Autodesk Inventor part; units mm, degrees
(part 2 of 7)
  line L132 (47.0881, -59.4916) -> (33.6537, -59.4916)
  arc A151 (44.1532, -52.5346) -> (44.1532, -56.5346) centre (44.1532, -54.5346) ccw
  line L133 (57.5876, -52.5346) -> (44.1532, -52.5346)
  arc A152 (57.5876, -56.5346) -> (57.5876, -52.5346) centre (57.5876, -54.5346) ccw
  line L134 (44.1532, -56.5346) -> (57.5876, -56.5346)
  line L135 (13.6537, -63.4916) -> (27.0881, -63.4916)
  line L136 (27.0881, -59.4916) -> (13.6537, -59.4916)
  arc A153 (24.1532, -52.5346) -> (24.1532, -56.5346) centre (24.1532, -54.5346) ccw
  arc A154 (27.0881, -63.4916) -> (27.0881, -59.4916) centre (27.0881, -61.4916) ccw
  arc A155 (33.6537, -59.4916) -> (33.6537, -63.4916) centre (33.6537, -61.4916) ccw
  line L137 (37.5876, -52.5346) -> (24.1532, -52.5346)
  line L138 (24.1532, -56.5346) -> (37.5876, -56.5346)
  arc A156 (37.5876, -56.5346) -> (37.5876, -52.5346) centre (37.5876, -54.5346) ccw
  line L139 (33.6537, -63.4916) -> (47.0881, -63.4916)
  arc A157 (-6.3463, -59.4916) -> (-6.3463, -63.4916) centre (-6.3463, -61.4916) ccw
  arc A158 (27.0881, -63.4916) -> (27.0881, -59.4916) centre (27.0881, -61.4916) ccw
  arc A159 (24.1532, -52.5346) -> (24.1532, -56.5346) centre (24.1532, -54.5346) ccw
  line L140 (27.0881, -59.4916) -> (13.6537, -59.4916)
  arc A160 (24.1532, -52.5346) -> (24.1532, -56.5346) centre (24.1532, -54.5346) ccw
  line L141 (37.5876, -52.5346) -> (24.1532, -52.5346)
  arc A161 (37.5876, -56.5346) -> (37.5876, -52.5346) centre (37.5876, -54.5346) ccw
  line L142 (24.1532, -56.5346) -> (37.5876, -56.5346)
  line L143 (-6.3463, -63.4916) -> (7.0881, -63.4916)
  line L144 (7.0881, -59.4916) -> (-6.3463, -59.4916)
  arc A162 (4.1532, -52.5346) -> (4.1532, -56.5346) centre (4.1532, -54.5346) ccw
  arc A163 (7.0881, -63.4916) -> (7.0881, -59.4916) centre (7.0881, -61.4916) ccw
  arc A164 (13.6537, -59.4916) -> (13.6537, -63.4916) centre (13.6537, -61.4916) ccw
  line L145 (17.5876, -52.5346) -> (4.1532, -52.5346)
  line L146 (4.1532, -56.5346) -> (17.5876, -56.5346)
  arc A165 (17.5876, -56.5346) -> (17.5876, -52.5346) centre (17.5876, -54.5346) ccw
  line L147 (13.6537, -63.4916) -> (27.0881, -63.4916)
  arc A166 (-26.3463, -59.4916) -> (-26.3463, -63.4916) centre (-26.3463, -61.4916) ccw
  arc A167 (7.0881, -63.4916) -> (7.0881, -59.4916) centre (7.0881, -61.4916) ccw
  arc A168 (4.1532, -52.5346) -> (4.1532, -56.5346) centre (4.1532, -54.5346) ccw
  line L148 (7.0881, -59.4916) -> (-6.3463, -59.4916)
  arc A169 (4.1532, -52.5346) -> (4.1532, -56.5346) centre (4.1532, -54.5346) ccw
  line L149 (17.5876, -52.5346) -> (4.1532, -52.5346)
  arc A170 (17.5876, -56.5346) -> (17.5876, -52.5346) centre (17.5876, -54.5346) ccw
  line L150 (4.1532, -56.5346) -> (17.5876, -56.5346)
  line L151 (-26.3463, -63.4916) -> (-12.9119, -63.4916)
  line L152 (-12.9119, -59.4916) -> (-26.3463, -59.4916)
  arc A171 (-15.8468, -52.5346) -> (-15.8468, -56.5346) centre (-15.8468, -54.5346) ccw
  arc A172 (-12.9119, -63.4916) -> (-12.9119, -59.4916) centre (-12.9119, -61.4916) ccw
  arc A173 (-6.3463, -59.4916) -> (-6.3463, -63.4916) centre (-6.3463, -61.4916) ccw
  line L153 (-2.4124, -52.5346) -> (-15.8468, -52.5346)
  line L154 (-15.8468, -56.5346) -> (-2.4124, -56.5346)
  arc A174 (-2.4124, -56.5346) -> (-2.4124, -52.5346) centre (-2.4124, -54.5346) ccw
  line L155 (-6.3463, -63.4916) -> (7.0881, -63.4916)
  arc A175 (-46.3463, -59.4916) -> (-46.3463, -63.4916) centre (-46.3463, -61.4916) ccw
  arc A176 (-12.9119, -63.4916) -> (-12.9119, -59.4916) centre (-12.9119, -61.4916) ccw
  arc A177 (-15.8468, -52.5346) -> (-15.8468, -56.5346) centre (-15.8468, -54.5346) ccw
  line L156 (-12.9119, -59.4916) -> (-26.3463, -59.4916)
  arc A178 (-15.8468, -52.5346) -> (-15.8468, -56.5346) centre (-15.8468, -54.5346) ccw
  line L157 (-2.4124, -52.5346) -> (-15.8468, -52.5346)
  arc A179 (-2.4124, -56.5346) -> (-2.4124, -52.5346) centre (-2.4124, -54.5346) ccw
  line L158 (-15.8468, -56.5346) -> (-2.4124, -56.5346)
  line L159 (-46.3463, -63.4916) -> (-32.9119, -63.4916)
  line L160 (-32.9119, -59.4916) -> (-46.3463, -59.4916)
  arc A180 (-35.8468, -52.5346) -> (-35.8468, -56.5346) centre (-35.8468, -54.5346) ccw
  arc A181 (-32.9119, -63.4916) -> (-32.9119, -59.4916) centre (-32.9119, -61.4916) ccw
  arc A182 (-26.3463, -59.4916) -> (-26.3463, -63.4916) centre (-26.3463, -61.4916) ccw
  line L161 (-22.4124, -52.5346) -> (-35.8468, -52.5346)
  line L162 (-35.8468, -56.5346) -> (-22.4124, -56.5346)
  arc A183 (-22.4124, -56.5346) -> (-22.4124, -52.5346) centre (-22.4124, -54.5346) ccw
  line L163 (-26.3463, -63.4916) -> (-12.9119, -63.4916)
  arc A184 (-66.3463, -59.4916) -> (-66.3463, -63.4916) centre (-66.3463, -61.4916) ccw
  arc A185 (-32.9119, -63.4916) -> (-32.9119, -59.4916) centre (-32.9119, -61.4916) ccw
  arc A186 (-35.8468, -52.5346) -> (-35.8468, -56.5346) centre (-35.8468, -54.5346) ccw
  line L164 (-32.9119, -59.4916) -> (-46.3463, -59.4916)
  arc A187 (-35.8468, -52.5346) -> (-35.8468, -56.5346) centre (-35.8468, -54.5346) ccw
  line L165 (-22.4124, -52.5346) -> (-35.8468, -52.5346)
  arc A188 (-22.4124, -56.5346) -> (-22.4124, -52.5346) centre (-22.4124, -54.5346) ccw
  line L166 (-35.8468, -56.5346) -> (-22.4124, -56.5346)
  line L167 (-66.3463, -63.4916) -> (-52.9119, -63.4916)
  line L168 (-52.9119, -59.4916) -> (-66.3463, -59.4916)
  arc A189 (-55.8468, -52.5346) -> (-55.8468, -56.5346) centre (-55.8468, -54.5346) ccw
  arc A190 (-52.9119, -63.4916) -> (-52.9119, -59.4916) centre (-52.9119, -61.4916) ccw
  arc A191 (-46.3463, -59.4916) -> (-46.3463, -63.4916) centre (-46.3463, -61.4916) ccw
  line L169 (-42.4124, -52.5346) -> (-55.8468, -52.5346)
  line L170 (-55.8468, -56.5346) -> (-42.4124, -56.5346)
  arc A192 (-42.4124, -56.5346) -> (-42.4124, -52.5346) centre (-42.4124, -54.5346) ccw
  line L171 (-46.3463, -63.4916) -> (-32.9119, -63.4916)
  arc A193 (44.1532, -38.5346) -> (44.1532, -42.5346) centre (44.1532, -40.5346) ccw
  arc A194 (44.1532, -38.5346) -> (44.1532, -42.5346) centre (44.1532, -40.5346) ccw
  arc A195 (44.1532, -38.5346) -> (44.1532, -42.5346) centre (44.1532, -40.5346) ccw
  arc A196 (44.1532, -38.5346) -> (44.1532, -42.5346) centre (44.1532, -40.5346) ccw
  arc A197 (44.1532, -38.5346) -> (44.1532, -42.5346) centre (44.1532, -40.5346) ccw
  arc A198 (44.1532, -38.5346) -> (44.1532, -42.5346) centre (44.1532, -40.5346) ccw
  arc A199 (44.1532, -38.5346) -> (44.1532, -42.5346) centre (44.1532, -40.5346) ccw
  arc A200 (33.6537, -45.4916) -> (33.6537, -49.4916) centre (33.6537, -47.4916) ccw
  arc A201 (27.0881, -49.4916) -> (27.0881, -45.4916) centre (27.0881, -47.4916) ccw
  arc A202 (27.0881, -49.4916) -> (27.0881, -45.4916) centre (27.0881, -47.4916) ccw
  arc A203 (33.6537, -45.4916) -> (33.6537, -49.4916) centre (33.6537, -47.4916) ccw
  arc A204 (27.0881, -49.4916) -> (27.0881, -45.4916) centre (27.0881, -47.4916) ccw
  arc A205 (27.0881, -49.4916) -> (27.0881, -45.4916) centre (27.0881, -47.4916) ccw
  arc A206 (27.0881, -49.4916) -> (27.0881, -45.4916) centre (27.0881, -47.4916) ccw
  arc A207 (27.0881, -49.4916) -> (27.0881, -45.4916) centre (27.0881, -47.4916) ccw
  arc A208 (33.6537, -45.4916) -> (33.6537, -49.4916) centre (33.6537, -47.4916) ccw
  arc A209 (33.6537, -45.4916) -> (33.6537, -49.4916) centre (33.6537, -47.4916) ccw
  arc A210 (33.6537, -45.4916) -> (33.6537, -49.4916) centre (33.6537, -47.4916) ccw
  line L172 (24.1532, -42.5346) -> (37.5876, -42.5346)
  line L173 (37.5876, -38.5346) -> (24.1532, -38.5346)
  line L174 (24.1532, -42.5346) -> (37.5876, -42.5346)
  line L175 (24.1532, -42.5346) -> (37.5876, -42.5346)
  line L176 (24.1532, -42.5346) -> (37.5876, -42.5346)
  line L177 (24.1532, -42.5346) -> (37.5876, -42.5346)
  line L178 (24.1532, -42.5346) -> (37.5876, -42.5346)
  line L179 (37.5876, -38.5346) -> (24.1532, -38.5346)
  line L180 (37.5876, -38.5346) -> (24.1532, -38.5346)
  line L181 (37.5876, -38.5346) -> (24.1532, -38.5346)
  line L182 (37.5876, -38.5346) -> (24.1532, -38.5346)
  line L183 (37.5876, -38.5346) -> (24.1532, -38.5346)
  arc A211 (37.5876, -42.5346) -> (37.5876, -38.5346) centre (37.5876, -40.5346) ccw
  arc A212 (37.5876, -42.5346) -> (37.5876, -38.5346) centre (37.5876, -40.5346) ccw
  arc A213 (37.5876, -42.5346) -> (37.5876, -38.5346) centre (37.5876, -40.5346) ccw
  arc A214 (37.5876, -42.5346) -> (37.5876, -38.5346) centre (37.5876, -40.5346) ccw
  arc A215 (37.5876, -42.5346) -> (37.5876, -38.5346) centre (37.5876, -40.5346) ccw
  arc A216 (37.5876, -42.5346) -> (37.5876, -38.5346) centre (37.5876, -40.5346) ccw
  arc A217 (44.1532, -38.5346) -> (44.1532, -42.5346) centre (44.1532, -40.5346) ccw
  arc A218 (47.0881, -49.4916) -> (47.0881, -45.4916) centre (47.0881, -47.4916) ccw
  arc A219 (47.0881, -49.4916) -> (47.0881, -45.4916) centre (47.0881, -47.4916) ccw
  arc A220 (53.6537, -45.4916) -> (53.6537, -49.4916) centre (53.6537, -47.4916) ccw
  arc A221 (47.0881, -49.4916) -> (47.0881, -45.4916) centre (47.0881, -47.4916) ccw
  arc A222 (47.0881, -49.4916) -> (47.0881, -45.4916) centre (47.0881, -47.4916) ccw
  arc A223 (47.0881, -49.4916) -> (47.0881, -45.4916) centre (47.0881, -47.4916) ccw
  arc A224 (53.6537, -45.4916) -> (53.6537, -49.4916) centre (53.6537, -47.4916) ccw
  arc A225 (53.6537, -45.4916) -> (53.6537, -49.4916) centre (53.6537, -47.4916) ccw
  line L184 (57.5876, -38.5346) -> (44.1532, -38.5346)
  line L185 (44.1532, -42.5346) -> (57.5876, -42.5346)
  line L186 (57.5876, -38.5346) -> (44.1532, -38.5346)
  line L187 (44.1532, -42.5346) -> (57.5876, -42.5346)
  line L188 (44.1532, -42.5346) -> (57.5876, -42.5346)
  line L189 (44.1532, -42.5346) -> (57.5876, -42.5346)
  line L190 (44.1532, -42.5346) -> (57.5876, -42.5346)
  line L191 (57.5876, -38.5346) -> (44.1532, -38.5346)
  line L192 (57.5876, -38.5346) -> (44.1532, -38.5346)
  line L193 (57.5876, -38.5346) -> (44.1532, -38.5346)
  arc A226 (57.5876, -42.5346) -> (57.5876, -38.5346) centre (57.5876, -40.5346) ccw
  arc A227 (64.1532, -38.5346) -> (64.1532, -42.5346) centre (64.1532, -40.5346) ccw
  line L194 (53.6537, -49.4916) -> (67.0881, -49.4916)
  line L195 (53.6537, -49.4916) -> (67.0881, -49.4916)
  line L196 (53.6537, -49.4916) -> (67.0881, -49.4916)
  line L197 (67.0881, -45.4916) -> (53.6537, -45.4916)
  line L198 (67.0881, -45.4916) -> (53.6537, -45.4916)
  line L199 (67.0881, -45.4916) -> (53.6537, -45.4916)
  arc A228 (64.1532, -38.5346) -> (64.1532, -42.5346) centre (64.1532, -40.5346) ccw
  arc A229 (64.1532, -38.5346) -> (64.1532, -42.5346) centre (64.1532, -40.5346) ccw
  arc A230 (64.1532, -38.5346) -> (64.1532, -42.5346) centre (64.1532, -40.5346) ccw
  arc A231 (64.1532, -38.5346) -> (64.1532, -42.5346) centre (64.1532, -40.5346) ccw
  arc A232 (57.5876, -42.5346) -> (57.5876, -38.5346) centre (57.5876, -40.5346) ccw
  arc A233 (57.5876, -42.5346) -> (57.5876, -38.5346) centre (57.5876, -40.5346) ccw
  arc A234 (57.5876, -42.5346) -> (57.5876, -38.5346) centre (57.5876, -40.5346) ccw
  arc A235 (57.5876, -42.5346) -> (57.5876, -38.5346) centre (57.5876, -40.5346) ccw
  arc A236 (67.0881, -49.4916) -> (67.0881, -45.4916) centre (67.0881, -47.4916) ccw
  arc A237 (67.0881, -49.4916) -> (67.0881, -45.4916) centre (67.0881, -47.4916) ccw
  arc A238 (67.0881, -49.4916) -> (67.0881, -45.4916) centre (67.0881, -47.4916) ccw
  line L200 (77.5876, -38.5346) -> (64.1532, -38.5346)
  line L201 (77.5876, -38.5346) -> (64.1532, -38.5346)
  line L202 (77.5876, -38.5346) -> (64.1532, -38.5346)
  line L203 (64.1532, -42.5346) -> (77.5876, -42.5346)
  line L204 (64.1532, -42.5346) -> (77.5876, -42.5346)
  line L205 (64.1532, -42.5346) -> (77.5876, -42.5346)
  arc A239 (73.6537, -45.4916) -> (73.6537, -49.4916) centre (73.6537, -47.4916) ccw
  arc A240 (77.5876, -42.5346) -> (77.5876, -38.5346) centre (77.5876, -40.5346) ccw
  arc A241 (77.5876, -42.5346) -> (77.5876, -38.5346) centre (77.5876, -40.5346) ccw
  arc A242 (77.5876, -42.5346) -> (77.5876, -38.5346) centre (77.5876, -40.5346) ccw
  arc A243 (84.1532, -38.5346) -> (84.1532, -42.5346) centre (84.1532, -40.5346) ccw
  arc A244 (84.1532, -38.5346) -> (84.1532, -42.5346) centre (84.1532, -40.5346) ccw
  line L206 (87.0881, -45.4916) -> (73.6537, -45.4916)
  arc A245 (87.0881, -49.4916) -> (87.0881, -45.4916) centre (87.0881, -47.4916) ccw
  line L207 (73.6537, -49.4916) -> (87.0881, -49.4916)
  line L208 (84.1532, -42.5346) -> (97.5876, -42.5346)
  line L209 (97.5876, -38.5346) -> (84.1532, -38.5346)
  arc A246 (97.5876, -42.5346) -> (97.5876, -38.5346) centre (97.5876, -40.5346) ccw
  line L210 (33.6537, -49.4916) -> (47.0881, -49.4916)
  line L211 (47.0881, -45.4916) -> (33.6537, -45.4916)
  line L212 (33.6537, -49.4916) -> (47.0881, -49.4916)
  line L213 (47.0881, -45.4916) -> (33.6537, -45.4916)
  line L214 (47.0881, -45.4916) -> (33.6537, -45.4916)
  line L215 (47.0881, -45.4916) -> (33.6537, -45.4916)
  line L216 (47.0881, -45.4916) -> (33.6537, -45.4916)
  line L217 (33.6537, -49.4916) -> (47.0881, -49.4916)
  line L218 (33.6537, -49.4916) -> (47.0881, -49.4916)
  line L219 (33.6537, -49.4916) -> (47.0881, -49.4916)
  arc A247 (13.6537, -45.4916) -> (13.6537, -49.4916) centre (13.6537, -47.4916) ccw
  arc A248 (13.6537, -45.4916) -> (13.6537, -49.4916) centre (13.6537, -47.4916) ccw
  arc A249 (13.6537, -45.4916) -> (13.6537, -49.4916) centre (13.6537, -47.4916) ccw
  arc A250 (13.6537, -45.4916) -> (13.6537, -49.4916) centre (13.6537, -47.4916) ccw
  arc A251 (13.6537, -45.4916) -> (13.6537, -49.4916) centre (13.6537, -47.4916) ccw
  arc A252 (13.6537, -45.4916) -> (13.6537, -49.4916) centre (13.6537, -47.4916) ccw
  arc A253 (7.0881, -49.4916) -> (7.0881, -45.4916) centre (7.0881, -47.4916) ccw
  arc A254 (7.0881, -49.4916) -> (7.0881, -45.4916) centre (7.0881, -47.4916) ccw
  arc A255 (7.0881, -49.4916) -> (7.0881, -45.4916) centre (7.0881, -47.4916) ccw
  arc A256 (7.0881, -49.4916) -> (7.0881, -45.4916) centre (7.0881, -47.4916) ccw
  arc A257 (17.5876, -42.5346) -> (17.5876, -38.5346) centre (17.5876, -40.5346) ccw
  arc A258 (17.5876, -42.5346) -> (17.5876, -38.5346) centre (17.5876, -40.5346) ccw
  arc A259 (17.5876, -42.5346) -> (17.5876, -38.5346) centre (17.5876, -40.5346) ccw
  arc A260 (17.5876, -42.5346) -> (17.5876, -38.5346) centre (17.5876, -40.5346) ccw
  arc A261 (17.5876, -42.5346) -> (17.5876, -38.5346) centre (17.5876, -40.5346) ccw
  arc A262 (17.5876, -42.5346) -> (17.5876, -38.5346) centre (17.5876, -40.5346) ccw
  arc A263 (24.1532, -38.5346) -> (24.1532, -42.5346) centre (24.1532, -40.5346) ccw
  arc A264 (24.1532, -38.5346) -> (24.1532, -42.5346) centre (24.1532, -40.5346) ccw
  arc A265 (24.1532, -38.5346) -> (24.1532, -42.5346) centre (24.1532, -40.5346) ccw
  arc A266 (24.1532, -38.5346) -> (24.1532, -42.5346) centre (24.1532, -40.5346) ccw
  arc A267 (24.1532, -38.5346) -> (24.1532, -42.5346) centre (24.1532, -40.5346) ccw
  arc A268 (24.1532, -38.5346) -> (24.1532, -42.5346) centre (24.1532, -40.5346) ccw
  arc A269 (24.1532, -38.5346) -> (24.1532, -42.5346) centre (24.1532, -40.5346) ccw
  arc A270 (24.1532, -38.5346) -> (24.1532, -42.5346) centre (24.1532, -40.5346) ccw
  arc A271 (24.1532, -38.5346) -> (24.1532, -42.5346) centre (24.1532, -40.5346) ccw
  arc A272 (4.1532, -38.5346) -> (4.1532, -42.5346) centre (4.1532, -40.5346) ccw
  arc A273 (4.1532, -38.5346) -> (4.1532, -42.5346) centre (4.1532, -40.5346) ccw
  arc A274 (4.1532, -38.5346) -> (4.1532, -42.5346) centre (4.1532, -40.5346) ccw
  arc A275 (4.1532, -38.5346) -> (4.1532, -42.5346) centre (4.1532, -40.5346) ccw
  arc A276 (4.1532, -38.5346) -> (4.1532, -42.5346) centre (4.1532, -40.5346) ccw
  arc A277 (4.1532, -38.5346) -> (4.1532, -42.5346) centre (4.1532, -40.5346) ccw
  arc A278 (4.1532, -38.5346) -> (4.1532, -42.5346) centre (4.1532, -40.5346) ccw
  arc A279 (4.1532, -38.5346) -> (4.1532, -42.5346) centre (4.1532, -40.5346) ccw
  arc A280 (4.1532, -38.5346) -> (4.1532, -42.5346) centre (4.1532, -40.5346) ccw
  arc A281 (-2.4124, -42.5346) -> (-2.4124, -38.5346) centre (-2.4124, -40.5346) ccw
  arc A282 (-2.4124, -42.5346) -> (-2.4124, -38.5346) centre (-2.4124, -40.5346) ccw
  arc A283 (-2.4124, -42.5346) -> (-2.4124, -38.5346) centre (-2.4124, -40.5346) ccw
  arc A284 (-2.4124, -42.5346) -> (-2.4124, -38.5346) centre (-2.4124, -40.5346) ccw
  arc A285 (-32.9119, -49.4916) -> (-32.9119, -45.4916) centre (-32.9119, -47.4916) ccw
  arc A286 (-32.9119, -49.4916) -> (-32.9119, -45.4916) centre (-32.9119, -47.4916) ccw
  arc A287 (-32.9119, -49.4916) -> (-32.9119, -45.4916) centre (-32.9119, -47.4916) ccw
  arc A288 (-32.9119, -49.4916) -> (-32.9119, -45.4916) centre (-32.9119, -47.4916) ccw
  arc A289 (-32.9119, -49.4916) -> (-32.9119, -45.4916) centre (-32.9119, -47.4916) ccw
  arc A290 (-32.9119, -49.4916) -> (-32.9119, -45.4916) centre (-32.9119, -47.4916) ccw
  line L220 (27.0881, -45.4916) -> (13.6537, -45.4916)
  line L221 (13.6537, -49.4916) -> (27.0881, -49.4916)
  line L222 (27.0881, -45.4916) -> (13.6537, -45.4916)
  line L223 (13.6537, -49.4916) -> (27.0881, -49.4916)
  line L224 (13.6537, -49.4916) -> (27.0881, -49.4916)
  line L225 (27.0881, -45.4916) -> (13.6537, -45.4916)
  line L226 (27.0881, -45.4916) -> (13.6537, -45.4916)
  line L227 (27.0881, -45.4916) -> (13.6537, -45.4916)
  line L228 (13.6537, -49.4916) -> (27.0881, -49.4916)
  line L229 (13.6537, -49.4916) -> (27.0881, -49.4916)
  line L230 (13.6537, -49.4916) -> (27.0881, -49.4916)
  line L231 (27.0881, -45.4916) -> (13.6537, -45.4916)
  line L232 (4.1532, -42.5346) -> (17.5876, -42.5346)
  line L233 (4.1532, -42.5346) -> (17.5876, -42.5346)
  line L234 (4.1532, -42.5346) -> (17.5876, -42.5346)
  line L235 (4.1532, -42.5346) -> (17.5876, -42.5346)
  line L236 (4.1532, -42.5346) -> (17.5876, -42.5346)
  line L237 (4.1532, -42.5346) -> (17.5876, -42.5346)
  line L238 (17.5876, -38.5346) -> (4.1532, -38.5346)
  line L239 (17.5876, -38.5346) -> (4.1532, -38.5346)
  line L240 (17.5876, -38.5346) -> (4.1532, -38.5346)
  line L241 (17.5876, -38.5346) -> (4.1532, -38.5346)
  line L242 (17.5876, -38.5346) -> (4.1532, -38.5346)
  line L243 (17.5876, -38.5346) -> (4.1532, -38.5346)
  arc A291 (7.0881, -49.4916) -> (7.0881, -45.4916) centre (7.0881, -47.4916) ccw
  arc A292 (7.0881, -49.4916) -> (7.0881, -45.4916) centre (7.0881, -47.4916) ccw
  line L244 (-6.3463, -49.4916) -> (7.0881, -49.4916)
  line L245 (7.0881, -45.4916) -> (-6.3463, -45.4916)
  line L246 (7.0881, -45.4916) -> (-6.3463, -45.4916)
  line L247 (-6.3463, -49.4916) -> (7.0881, -49.4916)
  line L248 (-6.3463, -49.4916) -> (7.0881, -49.4916)
  line L249 (7.0881, -45.4916) -> (-6.3463, -45.4916)
  line L250 (7.0881, -45.4916) -> (-6.3463, -45.4916)
  line L251 (7.0881, -45.4916) -> (-6.3463, -45.4916)
  line L252 (-6.3463, -49.4916) -> (7.0881, -49.4916)
  line L253 (-6.3463, -49.4916) -> (7.0881, -49.4916)
  line L254 (-6.3463, -49.4916) -> (7.0881, -49.4916)
  line L255 (7.0881, -45.4916) -> (-6.3463, -45.4916)
  arc A293 (-6.3463, -45.4916) -> (-6.3463, -49.4916) centre (-6.3463, -47.4916) ccw
  arc A294 (-6.3463, -45.4916) -> (-6.3463, -49.4916) centre (-6.3463, -47.4916) ccw
  arc A295 (-6.3463, -45.4916) -> (-6.3463, -49.4916) centre (-6.3463, -47.4916) ccw
  arc A296 (-6.3463, -45.4916) -> (-6.3463, -49.4916) centre (-6.3463, -47.4916) ccw
  arc A297 (-6.3463, -45.4916) -> (-6.3463, -49.4916) centre (-6.3463, -47.4916) ccw
  arc A298 (-6.3463, -45.4916) -> (-6.3463, -49.4916) centre (-6.3463, -47.4916) ccw
  arc A299 (-12.9119, -49.4916) -> (-12.9119, -45.4916) centre (-12.9119, -47.4916) ccw
  arc A300 (-12.9119, -49.4916) -> (-12.9119, -45.4916) centre (-12.9119, -47.4916) ccw
  arc A301 (-12.9119, -49.4916) -> (-12.9119, -45.4916) centre (-12.9119, -47.4916) ccw
  arc A302 (-12.9119, -49.4916) -> (-12.9119, -45.4916) centre (-12.9119, -47.4916) ccw
  arc A303 (-12.9119, -49.4916) -> (-12.9119, -45.4916) centre (-12.9119, -47.4916) ccw
  line L256 (-2.4124, -38.5346) -> (-15.8468, -38.5346)
  line L257 (-15.8468, -42.5346) -> (-2.4124, -42.5346)
  line L258 (-2.4124, -38.5346) -> (-15.8468, -38.5346)
  line L259 (-15.8468, -42.5346) -> (-2.4124, -42.5346)
  line L260 (-2.4124, -38.5346) -> (-15.8468, -38.5346)
  line L261 (-15.8468, -42.5346) -> (-2.4124, -42.5346)
  line L262 (-2.4124, -38.5346) -> (-15.8468, -38.5346)
  line L263 (-15.8468, -42.5346) -> (-2.4124, -42.5346)
  line L264 (-2.4124, -38.5346) -> (-15.8468, -38.5346)
  line L265 (-15.8468, -42.5346) -> (-2.4124, -42.5346)
  line L266 (-15.8468, -42.5346) -> (-2.4124, -42.5346)
  line L267 (-2.4124, -38.5346) -> (-15.8468, -38.5346)
  arc A304 (-2.4124, -42.5346) -> (-2.4124, -38.5346) centre (-2.4124, -40.5346) ccw
  arc A305 (-2.4124, -42.5346) -> (-2.4124, -38.5346) centre (-2.4124, -40.5346) ccw
  arc A306 (-15.8468, -38.5346) -> (-15.8468, -42.5346) centre (-15.8468, -40.5346) ccw
  arc A307 (-15.8468, -38.5346) -> (-15.8468, -42.5346) centre (-15.8468, -40.5346) ccw
  arc A308 (-15.8468, -38.5346) -> (-15.8468, -42.5346) centre (-15.8468, -40.5346) ccw
  arc A309 (-15.8468, -38.5346) -> (-15.8468, -42.5346) centre (-15.8468, -40.5346) ccw
  arc A310 (-15.8468, -38.5346) -> (-15.8468, -42.5346) centre (-15.8468, -40.5346) ccw
  arc A311 (-22.4124, -42.5346) -> (-22.4124, -38.5346) centre (-22.4124, -40.5346) ccw
  arc A312 (-22.4124, -42.5346) -> (-22.4124, -38.5346) centre (-22.4124, -40.5346) ccw
  arc A313 (-15.8468, -38.5346) -> (-15.8468, -42.5346) centre (-15.8468, -40.5346) ccw
  arc A314 (-15.8468, -38.5346) -> (-15.8468, -42.5346) centre (-15.8468, -40.5346) ccw
  arc A315 (-22.4124, -42.5346) -> (-22.4124, -38.5346) centre (-22.4124, -40.5346) ccw
  arc A316 (-15.8468, -38.5346) -> (-15.8468, -42.5346) centre (-15.8468, -40.5346) ccw
  arc A317 (-15.8468, -38.5346) -> (-15.8468, -42.5346) centre (-15.8468, -40.5346) ccw
  arc A318 (-22.4124, -42.5346) -> (-22.4124, -38.5346) centre (-22.4124, -40.5346) ccw
  arc A319 (-22.4124, -42.5346) -> (-22.4124, -38.5346) centre (-22.4124, -40.5346) ccw
  arc A320 (-22.4124, -42.5346) -> (-22.4124, -38.5346) centre (-22.4124, -40.5346) ccw
  arc A321 (-26.3463, -45.4916) -> (-26.3463, -49.4916) centre (-26.3463, -47.4916) ccw
  arc A322 (-26.3463, -45.4916) -> (-26.3463, -49.4916) centre (-26.3463, -47.4916) ccw
  arc A323 (-26.3463, -45.4916) -> (-26.3463, -49.4916) centre (-26.3463, -47.4916) ccw
  arc A324 (-26.3463, -45.4916) -> (-26.3463, -49.4916) centre (-26.3463, -47.4916) ccw
  arc A325 (-26.3463, -45.4916) -> (-26.3463, -49.4916) centre (-26.3463, -47.4916) ccw
  arc A326 (-26.3463, -45.4916) -> (-26.3463, -49.4916) centre (-26.3463, -47.4916) ccw
  line L268 (-35.8468, -42.5346) -> (-22.4124, -42.5346)
  line L269 (-35.8468, -42.5346) -> (-22.4124, -42.5346)
  line L270 (-35.8468, -42.5346) -> (-22.4124, -42.5346)
  line L271 (-35.8468, -42.5346) -> (-22.4124, -42.5346)
  line L272 (-35.8468, -42.5346) -> (-22.4124, -42.5346)
  line L273 (-35.8468, -42.5346) -> (-22.4124, -42.5346)
  line L274 (-22.4124, -38.5346) -> (-35.8468, -38.5346)
  line L275 (-22.4124, -38.5346) -> (-35.8468, -38.5346)
  line L276 (-22.4124, -38.5346) -> (-35.8468, -38.5346)
  line L277 (-22.4124, -38.5346) -> (-35.8468, -38.5346)
  line L278 (-22.4124, -38.5346) -> (-35.8468, -38.5346)
  line L279 (-22.4124, -38.5346) -> (-35.8468, -38.5346)
  line L280 (-26.3463, -49.4916) -> (-12.9119, -49.4916)
  line L281 (-12.9119, -45.4916) -> (-26.3463, -45.4916)
  line L282 (-12.9119, -45.4916) -> (-26.3463, -45.4916)
  line L283 (-26.3463, -49.4916) -> (-12.9119, -49.4916)
  line L284 (-12.9119, -45.4916) -> (-26.3463, -45.4916)
  line L285 (-12.9119, -45.4916) -> (-26.3463, -45.4916)
  line L286 (-26.3463, -49.4916) -> (-12.9119, -49.4916)
  line L287 (-12.9119, -45.4916) -> (-26.3463, -45.4916)
  line L288 (-12.9119, -45.4916) -> (-26.3463, -45.4916)
  line L289 (-26.3463, -49.4916) -> (-12.9119, -49.4916)
  line L290 (-26.3463, -49.4916) -> (-12.9119, -49.4916)
  line L291 (-26.3463, -49.4916) -> (-12.9119, -49.4916)
  arc A327 (-12.9119, -49.4916) -> (-12.9119, -45.4916) centre (-12.9119, -47.4916) ccw
  arc A328 (-46.3463, -45.4916) -> (-46.3463, -49.4916) centre (-46.3463, -47.4916) ccw
  arc A329 (-52.9119, -49.4916) -> (-52.9119, -45.4916) centre (-52.9119, -47.4916) ccw
  arc A330 (-46.3463, -45.4916) -> (-46.3463, -49.4916) centre (-46.3463, -47.4916) ccw
  arc A331 (-46.3463, -45.4916) -> (-46.3463, -49.4916) centre (-46.3463, -47.4916) ccw
  arc A332 (-46.3463, -45.4916) -> (-46.3463, -49.4916) centre (-46.3463, -47.4916) ccw
  arc A333 (-46.3463, -45.4916) -> (-46.3463, -49.4916) centre (-46.3463, -47.4916) ccw
  arc A334 (-46.3463, -45.4916) -> (-46.3463, -49.4916) centre (-46.3463, -47.4916) ccw
  arc A335 (-52.9119, -49.4916) -> (-52.9119, -45.4916) centre (-52.9119, -47.4916) ccw
  arc A336 (-52.9119, -49.4916) -> (-52.9119, -45.4916) centre (-52.9119, -47.4916) ccw
  arc A337 (-52.9119, -49.4916) -> (-52.9119, -45.4916) centre (-52.9119, -47.4916) ccw
  arc A338 (-52.9119, -49.4916) -> (-52.9119, -45.4916) centre (-52.9119, -47.4916) ccw
  line L292 (-42.4124, -38.5346) -> (-55.8468, -38.5346)
  line L293 (-55.8468, -42.5346) -> (-42.4124, -42.5346)
  line L294 (-55.8468, -42.5346) -> (-42.4124, -42.5346)
  line L295 (-55.8468, -42.5346) -> (-42.4124, -42.5346)
  line L296 (-55.8468, -42.5346) -> (-42.4124, -42.5346)
  line L297 (-55.8468, -42.5346) -> (-42.4124, -42.5346)
  line L298 (-42.4124, -38.5346) -> (-55.8468, -38.5346)
  line L299 (-42.4124, -38.5346) -> (-55.8468, -38.5346)
  line L300 (-42.4124, -38.5346) -> (-55.8468, -38.5346)
  line L301 (-42.4124, -38.5346) -> (-55.8468, -38.5346)
  arc A339 (-86.3463, -45.4916) -> (-86.3463, -49.4916) centre (-86.3463, -47.4916) ccw
  arc A340 (-86.3463, -45.4916) -> (-86.3463, -49.4916) centre (-86.3463, -47.4916) ccw
  arc A341 (-86.3463, -45.4916) -> (-86.3463, -49.4916) centre (-86.3463, -47.4916) ccw
  arc A342 (-92.9119, -49.4916) -> (-92.9119, -45.4916) centre (-92.9119, -47.4916) ccw
  line L302 (-82.4124, -38.5346) -> (-95.8468, -38.5346)
  line L303 (-95.8468, -42.5346) -> (-82.4124, -42.5346)
  line L304 (-86.3463, -49.4916) -> (-72.9119, -49.4916)
  line L305 (-86.3463, -49.4916) -> (-72.9119, -49.4916)
  line L306 (-86.3463, -49.4916) -> (-72.9119, -49.4916)
  line L307 (-72.9119, -45.4916) -> (-86.3463, -45.4916)
  line L308 (-72.9119, -45.4916) -> (-86.3463, -45.4916)
  line L309 (-72.9119, -45.4916) -> (-86.3463, -45.4916)
  arc A343 (-75.8468, -38.5346) -> (-75.8468, -42.5346) centre (-75.8468, -40.5346) ccw
  arc A344 (-75.8468, -38.5346) -> (-75.8468, -42.5346) centre (-75.8468, -40.5346) ccw
  arc A345 (-75.8468, -38.5346) -> (-75.8468, -42.5346) centre (-75.8468, -40.5346) ccw
  arc A346 (-75.8468, -38.5346) -> (-75.8468, -42.5346) centre (-75.8468, -40.5346) ccw
  arc A347 (-82.4124, -42.5346) -> (-82.4124, -38.5346) centre (-82.4124, -40.5346) ccw
  line L310 (-66.3463, -49.4916) -> (-52.9119, -49.4916)
  line L311 (-52.9119, -45.4916) -> (-66.3463, -45.4916)
  line L312 (-52.9119, -45.4916) -> (-66.3463, -45.4916)
  line L313 (-66.3463, -49.4916) -> (-52.9119, -49.4916)
  line L314 (-52.9119, -45.4916) -> (-66.3463, -45.4916)
  line L315 (-52.9119, -45.4916) -> (-66.3463, -45.4916)
  line L316 (-52.9119, -45.4916) -> (-66.3463, -45.4916)
  line L317 (-66.3463, -49.4916) -> (-52.9119, -49.4916)
  line L318 (-66.3463, -49.4916) -> (-52.9119, -49.4916)
  line L319 (-66.3463, -49.4916) -> (-52.9119, -49.4916)
  line L320 (-46.3463, -49.4916) -> (-32.9119, -49.4916)
  line L321 (-32.9119, -45.4916) -> (-46.3463, -45.4916)
  line L322 (-32.9119, -45.4916) -> (-46.3463, -45.4916)
  line L323 (-46.3463, -49.4916) -> (-32.9119, -49.4916)
  line L324 (-32.9119, -45.4916) -> (-46.3463, -45.4916)
  line L325 (-32.9119, -45.4916) -> (-46.3463, -45.4916)
  line L326 (-32.9119, -45.4916) -> (-46.3463, -45.4916)
  line L327 (-46.3463, -49.4916) -> (-32.9119, -49.4916)
  line L328 (-46.3463, -49.4916) -> (-32.9119, -49.4916)
  line L329 (-46.3463, -49.4916) -> (-32.9119, -49.4916)
  line L330 (-46.3463, -49.4916) -> (-32.9119, -49.4916)
  line L331 (-32.9119, -45.4916) -> (-46.3463, -45.4916)
  arc A348 (-55.8468, -38.5346) -> (-55.8468, -42.5346) centre (-55.8468, -40.5346) ccw
  arc A349 (-55.8468, -38.5346) -> (-55.8468, -42.5346) centre (-55.8468, -40.5346) ccw
  arc A350 (-55.8468, -38.5346) -> (-55.8468, -42.5346) centre (-55.8468, -40.5346) ccw
  arc A351 (-62.4124, -42.5346) -> (-62.4124, -38.5346) centre (-62.4124, -40.5346) ccw
  arc A352 (-55.8468, -38.5346) -> (-55.8468, -42.5346) centre (-55.8468, -40.5346) ccw
  arc A353 (-55.8468, -38.5346) -> (-55.8468, -42.5346) centre (-55.8468, -40.5346) ccw
  arc A354 (-55.8468, -38.5346) -> (-55.8468, -42.5346) centre (-55.8468, -40.5346) ccw
  arc A355 (-55.8468, -38.5346) -> (-55.8468, -42.5346) centre (-55.8468, -40.5346) ccw
  arc A356 (-62.4124, -42.5346) -> (-62.4124, -38.5346) centre (-62.4124, -40.5346) ccw
  arc A357 (-62.4124, -42.5346) -> (-62.4124, -38.5346) centre (-62.4124, -40.5346) ccw
  arc A358 (-66.3463, -45.4916) -> (-66.3463, -49.4916) centre (-66.3463, -47.4916) ccw
  arc A359 (-72.9119, -49.4916) -> (-72.9119, -45.4916) centre (-72.9119, -47.4916) ccw
  arc A360 (-66.3463, -45.4916) -> (-66.3463, -49.4916) centre (-66.3463, -47.4916) ccw
  line L332 (-62.4124, -38.5346) -> (-75.8468, -38.5346)
  line L333 (-75.8468, -42.5346) -> (-62.4124, -42.5346)
  arc A361 (-72.9119, -49.4916) -> (-72.9119, -45.4916) centre (-72.9119, -47.4916) ccw
  line L334 (-62.4124, -38.5346) -> (-75.8468, -38.5346)
  line L335 (-75.8468, -42.5346) -> (-62.4124, -42.5346)
  arc A362 (-66.3463, -45.4916) -> (-66.3463, -49.4916) centre (-66.3463, -47.4916) ccw
  arc A363 (-66.3463, -45.4916) -> (-66.3463, -49.4916) centre (-66.3463, -47.4916) ccw
  arc A364 (-66.3463, -45.4916) -> (-66.3463, -49.4916) centre (-66.3463, -47.4916) ccw
  line L336 (-62.4124, -38.5346) -> (-75.8468, -38.5346)
  line L337 (-75.8468, -42.5346) -> (-62.4124, -42.5346)
  arc A365 (-72.9119, -49.4916) -> (-72.9119, -45.4916) centre (-72.9119, -47.4916) ccw
  arc A366 (-106.3463, -45.4916) -> (-106.3463, -49.4916) centre (-106.3463, -47.4916) ccw
  arc A367 (-95.8468, -38.5346) -> (-95.8468, -42.5346) centre (-95.8468, -40.5346) ccw
  line L338 (-92.9119, -45.4916) -> (-106.3463, -45.4916)
  line L339 (-106.3463, -49.4916) -> (-92.9119, -49.4916)
  arc A368 (-35.8468, -38.5346) -> (-35.8468, -42.5346) centre (-35.8468, -40.5346) ccw
  arc A369 (-35.8468, -38.5346) -> (-35.8468, -42.5346) centre (-35.8468, -40.5346) ccw
  arc A370 (-35.8468, -38.5346) -> (-35.8468, -42.5346) centre (-35.8468, -40.5346) ccw
  arc A371 (-42.4124, -42.5346) -> (-42.4124, -38.5346) centre (-42.4124, -40.5346) ccw
  arc A372 (-42.4124, -42.5346) -> (-42.4124, -38.5346) centre (-42.4124, -40.5346) ccw
  arc A373 (-35.8468, -38.5346) -> (-35.8468, -42.5346) centre (-35.8468, -40.5346) ccw
  arc A374 (-35.8468, -38.5346) -> (-35.8468, -42.5346) centre (-35.8468, -40.5346) ccw
  arc A375 (-35.8468, -38.5346) -> (-35.8468, -42.5346) centre (-35.8468, -40.5346) ccw
  arc A376 (-35.8468, -38.5346) -> (-35.8468, -42.5346) centre (-35.8468, -40.5346) ccw
  arc A377 (-35.8468, -38.5346) -> (-35.8468, -42.5346) centre (-35.8468, -40.5346) ccw
  arc A378 (-35.8468, -38.5346) -> (-35.8468, -42.5346) centre (-35.8468, -40.5346) ccw
  arc A379 (-42.4124, -42.5346) -> (-42.4124, -38.5346) centre (-42.4124, -40.5346) ccw
  arc A380 (-42.4124, -42.5346) -> (-42.4124, -38.5346) centre (-42.4124, -40.5346) ccw
  arc A381 (-42.4124, -42.5346) -> (-42.4124, -38.5346) centre (-42.4124, -40.5346) ccw
  arc A382 (44.1532, -24.5346) -> (44.1532, -28.5346) centre (44.1532, -26.5346) ccw
  arc A383 (44.1532, -24.5346) -> (44.1532, -28.5346) centre (44.1532, -26.5346) ccw
  arc A384 (44.1532, -24.5346) -> (44.1532, -28.5346) centre (44.1532, -26.5346) ccw
  arc A385 (44.1532, -24.5346) -> (44.1532, -28.5346) centre (44.1532, -26.5346) ccw
  arc A386 (44.1532, -24.5346) -> (44.1532, -28.5346) centre (44.1532, -26.5346) ccw
  arc A387 (44.1532, -24.5346) -> (44.1532, -28.5346) centre (44.1532, -26.5346) ccw
  arc A388 (44.1532, -24.5346) -> (44.1532, -28.5346) centre (44.1532, -26.5346) ccw
  arc A389 (33.6537, -31.4916) -> (33.6537, -35.4916) centre (33.6537, -33.4916) ccw
  arc A390 (27.0881, -35.4916) -> (27.0881, -31.4916) centre (27.0881, -33.4916) ccw
  arc A391 (27.0881, -35.4916) -> (27.0881, -31.4916) centre (27.0881, -33.4916) ccw
  arc A392 (33.6537, -31.4916) -> (33.6537, -35.4916) centre (33.6537, -33.4916) ccw
  arc A393 (27.0881, -35.4916) -> (27.0881, -31.4916) centre (27.0881, -33.4916) ccw
  arc A394 (27.0881, -35.4916) -> (27.0881, -31.4916) centre (27.0881, -33.4916) ccw
  arc A395 (27.0881, -35.4916) -> (27.0881, -31.4916) centre (27.0881, -33.4916) ccw
  arc A396 (27.0881, -35.4916) -> (27.0881, -31.4916) centre (27.0881, -33.4916) ccw
  arc A397 (33.6537, -31.4916) -> (33.6537, -35.4916) centre (33.6537, -33.4916) ccw
  arc A398 (33.6537, -31.4916) -> (33.6537, -35.4916) centre (33.6537, -33.4916) ccw
  arc A399 (33.6537, -31.4916) -> (33.6537, -35.4916) centre (33.6537, -33.4916) ccw
  line L340 (24.1532, -28.5346) -> (37.5876, -28.5346)
  line L341 (37.5876, -24.5346) -> (24.1532, -24.5346)
  line L342 (24.1532, -28.5346) -> (37.5876, -28.5346)
  line L343 (24.1532, -28.5346) -> (37.5876, -28.5346)
  line L344 (24.1532, -28.5346) -> (37.5876, -28.5346)
  line L345 (24.1532, -28.5346) -> (37.5876, -28.5346)
  line L346 (24.1532, -28.5346) -> (37.5876, -28.5346)
  line L347 (37.5876, -24.5346) -> (24.1532, -24.5346)
  line L348 (37.5876, -24.5346) -> (24.1532, -24.5346)
  line L349 (37.5876, -24.5346) -> (24.1532, -24.5346)
  line L350 (37.5876, -24.5346) -> (24.1532, -24.5346)
  line L351 (37.5876, -24.5346) -> (24.1532, -24.5346)
  arc A400 (37.5876, -28.5346) -> (37.5876, -24.5346) centre (37.5876, -26.5346) ccw
  arc A401 (37.5876, -28.5346) -> (37.5876, -24.5346) centre (37.5876, -26.5346) ccw
  arc A402 (37.5876, -28.5346) -> (37.5876, -24.5346) centre (37.5876, -26.5346) ccw
  arc A403 (37.5876, -28.5346) -> (37.5876, -24.5346) centre (37.5876, -26.5346) ccw
  arc A404 (37.5876, -28.5346) -> (37.5876, -24.5346) centre (37.5876, -26.5346) ccw
  arc A405 (37.5876, -28.5346) -> (37.5876, -24.5346) centre (37.5876, -26.5346) ccw
  arc A406 (44.1532, -24.5346) -> (44.1532, -28.5346) centre (44.1532, -26.5346) ccw
  arc A407 (47.0881, -35.4916) -> (47.0881, -31.4916) centre (47.0881, -33.4916) ccw
  arc A408 (47.0881, -35.4916) -> (47.0881, -31.4916) centre (47.0881, -33.4916) ccw
  arc A409 (53.6537, -31.4916) -> (53.6537, -35.4916) centre (53.6537, -33.4916) ccw
  arc A410 (47.0881, -35.4916) -> (47.0881, -31.4916) centre (47.0881, -33.4916) ccw
  arc A411 (47.0881, -35.4916) -> (47.0881, -31.4916) centre (47.0881, -33.4916) ccw
  arc A412 (47.0881, -35.4916) -> (47.0881, -31.4916) centre (47.0881, -33.4916) ccw
  arc A413 (53.6537, -31.4916) -> (53.6537, -35.4916) centre (53.6537, -33.4916) ccw
  arc A414 (53.6537, -31.4916) -> (53.6537, -35.4916) centre (53.6537, -33.4916) ccw
  line L352 (57.5876, -24.5346) -> (44.1532, -24.5346)
  line L353 (44.1532, -28.5346) -> (57.5876, -28.5346)
  line L354 (57.5876, -24.5346) -> (44.1532, -24.5346)
  line L355 (44.1532, -28.5346) -> (57.5876, -28.5346)
  line L356 (44.1532, -28.5346) -> (57.5876, -28.5346)
  line L357 (44.1532, -28.5346) -> (57.5876, -28.5346)
  line L358 (44.1532, -28.5346) -> (57.5876, -28.5346)
  line L359 (57.5876, -24.5346) -> (44.1532, -24.5346)
  line L360 (57.5876, -24.5346) -> (44.1532, -24.5346)
  line L361 (57.5876, -24.5346) -> (44.1532, -24.5346)
  arc A415 (57.5876, -28.5346) -> (57.5876, -24.5346) centre (57.5876, -26.5346) ccw
  arc A416 (64.1532, -24.5346) -> (64.1532, -28.5346) centre (64.1532, -26.5346) ccw
  line L362 (53.6537, -35.4916) -> (67.0881, -35.4916)
  line L363 (53.6537, -35.4916) -> (67.0881, -35.4916)
  line L364 (53.6537, -35.4916) -> (67.0881, -35.4916)
  line L365 (67.0881, -31.4916) -> (53.6537, -31.4916)
  line L366 (67.0881, -31.4916) -> (53.6537, -31.4916)
  line L367 (67.0881, -31.4916) -> (53.6537, -31.4916)
  arc A417 (64.1532, -24.5346) -> (64.1532, -28.5346) centre (64.1532, -26.5346) ccw
  arc A418 (64.1532, -24.5346) -> (64.1532, -28.5346) centre (64.1532, -26.5346) ccw
  arc A419 (64.1532, -24.5346) -> (64.1532, -28.5346) centre (64.1532, -26.5346) ccw
  arc A420 (64.1532, -24.5346) -> (64.1532, -28.5346) centre (64.1532, -26.5346) ccw
  arc A421 (57.5876, -28.5346) -> (57.5876, -24.5346) centre (57.5876, -26.5346) ccw
  arc A422 (57.5876, -28.5346) -> (57.5876, -24.5346) centre (57.5876, -26.5346) ccw
  arc A423 (57.5876, -28.5346) -> (57.5876, -24.5346) centre (57.5876, -26.5346) ccw
  arc A424 (57.5876, -28.5346) -> (57.5876, -24.5346) centre (57.5876, -26.5346) ccw
  arc A425 (67.0881, -35.4916) -> (67.0881, -31.4916) centre (67.0881, -33.4916) ccw
  arc A426 (67.0881, -35.4916) -> (67.0881, -31.4916) centre (67.0881, -33.4916) ccw
  arc A427 (67.0881, -35.4916) -> (67.0881, -31.4916) centre (67.0881, -33.4916) ccw
  line L368 (77.5876, -24.5346) -> (64.1532, -24.5346)
  line L369 (77.5876, -24.5346) -> (64.1532, -24.5346)
  line L370 (77.5876, -24.5346) -> (64.1532, -24.5346)
  line L371 (64.1532, -28.5346) -> (77.5876, -28.5346)
  line L372 (64.1532, -28.5346) -> (77.5876, -28.5346)
  line L373 (64.1532, -28.5346) -> (77.5876, -28.5346)
  arc A428 (73.6537, -31.4916) -> (73.6537, -35.4916) centre (73.6537, -33.4916) ccw
  arc A429 (77.5876, -28.5346) -> (77.5876, -24.5346) centre (77.5876, -26.5346) ccw
  arc A430 (77.5876, -28.5346) -> (77.5876, -24.5346) centre (77.5876, -26.5346) ccw
  arc A431 (77.5876, -28.5346) -> (77.5876, -24.5346) centre (77.5876, -26.5346) ccw
  arc A432 (84.1532, -24.5346) -> (84.1532, -28.5346) centre (84.1532, -26.5346) ccw
  arc A433 (84.1532, -24.5346) -> (84.1532, -28.5346) centre (84.1532, -26.5346) ccw
  line L374 (87.0881, -31.4916) -> (73.6537, -31.4916)
  arc A434 (87.0881, -35.4916) -> (87.0881, -31.4916) centre (87.0881, -33.4916) ccw
  line L375 (73.6537, -35.4916) -> (87.0881, -35.4916)
  line L376 (84.1532, -28.5346) -> (97.5876, -28.5346)
  line L377 (97.5876, -24.5346) -> (84.1532, -24.5346)
  arc A435 (97.5876, -28.5346) -> (97.5876, -24.5346) centre (97.5876, -26.5346) ccw
  line L378 (33.6537, -35.4916) -> (47.0881, -35.4916)
  line L379 (47.0881, -31.4916) -> (33.6537, -31.4916)
  line L380 (33.6537, -35.4916) -> (47.0881, -35.4916)
  line L381 (47.0881, -31.4916) -> (33.6537, -31.4916)
  line L382 (47.0881, -31.4916) -> (33.6537, -31.4916)
  line L383 (47.0881, -31.4916) -> (33.6537, -31.4916)
  line L384 (47.0881, -31.4916) -> (33.6537, -31.4916)
  line L385 (33.6537, -35.4916) -> (47.0881, -35.4916)
  line L386 (33.6537, -35.4916) -> (47.0881, -35.4916)
  line L387 (33.6537, -35.4916) -> (47.0881, -35.4916)
  arc A436 (13.6537, -31.4916) -> (13.6537, -35.4916) centre (13.6537, -33.4916) ccw
  arc A437 (13.6537, -31.4916) -> (13.6537, -35.4916) centre (13.6537, -33.4916) ccw
  arc A438 (13.6537, -31.4916) -> (13.6537, -35.4916) centre (13.6537, -33.4916) ccw
  arc A439 (13.6537, -31.4916) -> (13.6537, -35.4916) centre (13.6537, -33.4916) ccw
  arc A440 (13.6537, -31.4916) -> (13.6537, -35.4916) centre (13.6537, -33.4916) ccw
  arc A441 (13.6537, -31.4916) -> (13.6537, -35.4916) centre (13.6537, -33.4916) ccw
  arc A442 (7.0881, -35.4916) -> (7.0881, -31.4916) centre (7.0881, -33.4916) ccw
  arc A443 (7.0881, -35.4916) -> (7.0881, -31.4916) centre (7.0881, -33.4916) ccw
  arc A444 (7.0881, -35.4916) -> (7.0881, -31.4916) centre (7.0881, -33.4916) ccw
  arc A445 (7.0881, -35.4916) -> (7.0881, -31.4916) centre (7.0881, -33.4916) ccw
  arc A446 (17.5876, -28.5346) -> (17.5876, -24.5346) centre (17.5876, -26.5346) ccw
  arc A447 (17.5876, -28.5346) -> (17.5876, -24.5346) centre (17.5876, -26.5346) ccw
  arc A448 (17.5876, -28.5346) -> (17.5876, -24.5346) centre (17.5876, -26.5346) ccw
  arc A449 (17.5876, -28.5346) -> (17.5876, -24.5346) centre (17.5876, -26.5346) ccw
  arc A450 (17.5876, -28.5346) -> (17.5876, -24.5346) centre (17.5876, -26.5346) ccw
  arc A451 (17.5876, -28.5346) -> (17.5876, -24.5346) centre (17.5876, -26.5346) ccw
  arc A452 (24.1532, -24.5346) -> (24.1532, -28.5346) centre (24.1532, -26.5346) ccw
  arc A453 (24.1532, -24.5346) -> (24.1532, -28.5346) centre (24.1532, -26.5346) ccw
  arc A454 (24.1532, -24.5346) -> (24.1532, -28.5346) centre (24.1532, -26.5346) ccw
  arc A455 (24.1532, -24.5346) -> (24.1532, -28.5346) centre (24.1532, -26.5346) ccw
  arc A456 (24.1532, -24.5346) -> (24.1532, -28.5346) centre (24.1532, -26.5346) ccw
  arc A457 (24.1532, -24.5346) -> (24.1532, -28.5346) centre (24.1532, -26.5346) ccw
  arc A458 (24.1532, -24.5346) -> (24.1532, -28.5346) centre (24.1532, -26.5346) ccw
  arc A459 (24.1532, -24.5346) -> (24.1532, -28.5346) centre (24.1532, -26.5346) ccw
  arc A460 (24.1532, -24.5346) -> (24.1532, -28.5346) centre (24.1532, -26.5346) ccw
  arc A461 (4.1532, -24.5346) -> (4.1532, -28.5346) centre (4.1532, -26.5346) ccw
  arc A462 (4.1532, -24.5346) -> (4.1532, -28.5346) centre (4.1532, -26.5346) ccw
  arc A463 (4.1532, -24.5346) -> (4.1532, -28.5346) centre (4.1532, -26.5346) ccw
  arc A464 (4.1532, -24.5346) -> (4.1532, -28.5346) centre (4.1532, -26.5346) ccw
  arc A465 (4.1532, -24.5346) -> (4.1532, -28.5346) centre (4.1532, -26.5346) ccw
  arc A466 (4.1532, -24.5346) -> (4.1532, -28.5346) centre (4.1532, -26.5346) ccw
  arc A467 (4.1532, -24.5346) -> (4.1532, -28.5346) centre (4.1532, -26.5346) ccw
  arc A468 (4.1532, -24.5346) -> (4.1532, -28.5346) centre (4.1532, -26.5346) ccw
  arc A469 (4.1532, -24.5346) -> (4.1532, -28.5346) centre (4.1532, -26.5346) ccw
  arc A470 (-2.4124, -28.5346) -> (-2.4124, -24.5346) centre (-2.4124, -26.5346) ccw
  arc A471 (-2.4124, -28.5346) -> (-2.4124, -24.5346) centre (-2.4124, -26.5346) ccw
  arc A472 (-2.4124, -28.5346) -> (-2.4124, -24.5346) centre (-2.4124, -26.5346) ccw
  arc A473 (-2.4124, -28.5346) -> (-2.4124, -24.5346) centre (-2.4124, -26.5346) ccw
  arc A474 (-32.9119, -35.4916) -> (-32.9119, -31.4916) centre (-32.9119, -33.4916) ccw
  arc A475 (-32.9119, -35.4916) -> (-32.9119, -31.4916) centre (-32.9119, -33.4916) ccw
  arc A476 (-32.9119, -35.4916) -> (-32.9119, -31.4916) centre (-32.9119, -33.4916) ccw
  arc A477 (-32.9119, -35.4916) -> (-32.9119, -31.4916) centre (-32.9119, -33.4916) ccw
  arc A478 (-32.9119, -35.4916) -> (-32.9119, -31.4916) centre (-32.9119, -33.4916) ccw
  arc A479 (-32.9119, -35.4916) -> (-32.9119, -31.4916) centre (-32.9119, -33.4916) ccw
  line L388 (27.0881, -31.4916) -> (13.6537, -31.4916)
  line L389 (13.6537, -35.4916) -> (27.0881, -35.4916)
  line L390 (27.0881, -31.4916) -> (13.6537, -31.4916)
  line L391 (13.6537, -35.4916) -> (27.0881, -35.4916)
  line L392 (13.6537, -35.4916) -> (27.0881, -35.4916)
  line L393 (27.0881, -31.4916) -> (13.6537, -31.4916)
  line L394 (27.0881, -31.4916) -> (13.6537, -31.4916)
  line L395 (27.0881, -31.4916) -> (13.6537, -31.4916)
  line L396 (13.6537, -35.4916) -> (27.0881, -35.4916)
  line L397 (13.6537, -35.4916) -> (27.0881, -35.4916)
  line L398 (13.6537, -35.4916) -> (27.0881, -35.4916)
  line L399 (27.0881, -31.4916) -> (13.6537, -31.4916)
  line L400 (4.1532, -28.5346) -> (17.5876, -28.5346)
  line L401 (4.1532, -28.5346) -> (17.5876, -28.5346)
  line L402 (4.1532, -28.5346) -> (17.5876, -28.5346)
  line L403 (4.1532, -28.5346) -> (17.5876, -28.5346)
  line L404 (4.1532, -28.5346) -> (17.5876, -28.5346)
  line L405 (4.1532, -28.5346) -> (17.5876, -28.5346)
  line L406 (17.5876, -24.5346) -> (4.1532, -24.5346)
  line L407 (17.5876, -24.5346) -> (4.1532, -24.5346)
  line L408 (17.5876, -24.5346) -> (4.1532, -24.5346)
  line L409 (17.5876, -24.5346) -> (4.1532, -24.5346)
  line L410 (17.5876, -24.5346) -> (4.1532, -24.5346)
  line L411 (17.5876, -24.5346) -> (4.1532, -24.5346)
  arc A480 (7.0881, -35.4916) -> (7.0881, -31.4916) centre (7.0881, -33.4916) ccw
  arc A481 (7.0881, -35.4916) -> (7.0881, -31.4916) centre (7.0881, -33.4916) ccw
  line L412 (-6.3463, -35.4916) -> (7.0881, -35.4916)
  line L413 (7.0881, -31.4916) -> (-6.3463, -31.4916)
  line L414 (7.0881, -31.4916) -> (-6.3463, -31.4916)
  line L415 (-6.3463, -35.4916) -> (7.0881, -35.4916)
  line L416 (-6.3463, -35.4916) -> (7.0881, -35.4916)
  line L417 (7.0881, -31.4916) -> (-6.3463, -31.4916)
  line L418 (7.0881, -31.4916) -> (-6.3463, -31.4916)
  line L419 (7.0881, -31.4916) -> (-6.3463, -31.4916)
  line L420 (-6.3463, -35.4916) -> (7.0881, -35.4916)
  line L421 (-6.3463, -35.4916) -> (7.0881, -35.4916)
  line L422 (-6.3463, -35.4916) -> (7.0881, -35.4916)
  line L423 (7.0881, -31.4916) -> (-6.3463, -31.4916)
  arc A482 (-6.3463, -31.4916) -> (-6.3463, -35.4916) centre (-6.3463, -33.4916) ccw
  arc A483 (-6.3463, -31.4916) -> (-6.3463, -35.4916) centre (-6.3463, -33.4916) ccw
  arc A484 (-6.3463, -31.4916) -> (-6.3463, -35.4916) centre (-6.3463, -33.4916) ccw
  arc A485 (-6.3463, -31.4916) -> (-6.3463, -35.4916) centre (-6.3463, -33.4916) ccw
  arc A486 (-6.3463, -31.4916) -> (-6.3463, -35.4916) centre (-6.3463, -33.4916) ccw
  arc A487 (-6.3463, -31.4916) -> (-6.3463, -35.4916) centre (-6.3463, -33.4916) ccw
  arc A488 (-12.9119, -35.4916) -> (-12.9119, -31.4916) centre (-12.9119, -33.4916) ccw
  arc A489 (-12.9119, -35.4916) -> (-12.9119, -31.4916) centre (-12.9119, -33.4916) ccw
  arc A490 (-12.9119, -35.4916) -> (-12.9119, -31.4916) centre (-12.9119, -33.4916) ccw
  arc A491 (-12.9119, -35.4916) -> (-12.9119, -31.4916) centre (-12.9119, -33.4916) ccw
  arc A492 (-12.9119, -35.4916) -> (-12.9119, -31.4916) centre (-12.9119, -33.4916) ccw
  line L424 (-2.4124, -24.5346) -> (-15.8468, -24.5346)
  line L425 (-15.8468, -28.5346) -> (-2.4124, -28.5346)
  line L426 (-2.4124, -24.5346) -> (-15.8468, -24.5346)
  line L427 (-15.8468, -28.5346) -> (-2.4124, -28.5346)
  line L428 (-2.4124, -24.5346) -> (-15.8468, -24.5346)
  line L429 (-15.8468, -28.5346) -> (-2.4124, -28.5346)
  line L430 (-2.4124, -24.5346) -> (-15.8468, -24.5346)
  line L431 (-15.8468, -28.5346) -> (-2.4124, -28.5346)
  line L432 (-2.4124, -24.5346) -> (-15.8468, -24.5346)
  line L433 (-15.8468, -28.5346) -> (-2.4124, -28.5346)
  line L434 (-15.8468, -28.5346) -> (-2.4124, -28.5346)
  line L435 (-2.4124, -24.5346) -> (-15.8468, -24.5346)
  arc A493 (-2.4124, -28.5346) -> (-2.4124, -24.5346) centre (-2.4124, -26.5346) ccw
  arc A494 (-2.4124, -28.5346) -> (-2.4124, -24.5346) centre (-2.4124, -26.5346) ccw
  arc A495 (-15.8468, -24.5346) -> (-15.8468, -28.5346) centre (-15.8468, -26.5346) ccw
  arc A496 (-15.8468, -24.5346) -> (-15.8468, -28.5346) centre (-15.8468, -26.5346) ccw
  arc A497 (-15.8468, -24.5346) -> (-15.8468, -28.5346) centre (-15.8468, -26.5346) ccw
  arc A498 (-15.8468, -24.5346) -> (-15.8468, -28.5346) centre (-15.8468, -26.5346) ccw
  arc A499 (-15.8468, -24.5346) -> (-15.8468, -28.5346) centre (-15.8468, -26.5346) ccw
  arc A500 (-22.4124, -28.5346) -> (-22.4124, -24.5346) centre (-22.4124, -26.5346) ccw
  arc A501 (-22.4124, -28.5346) -> (-22.4124, -24.5346) centre (-22.4124, -26.5346) ccw
  arc A502 (-15.8468, -24.5346) -> (-15.8468, -28.5346) centre (-15.8468, -26.5346) ccw
  arc A503 (-15.8468, -24.5346) -> (-15.8468, -28.5346) centre (-15.8468, -26.5346) ccw
  arc A504 (-22.4124, -28.5346) -> (-22.4124, -24.5346) centre (-22.4124, -26.5346) ccw
  arc A505 (-15.8468, -24.5346) -> (-15.8468, -28.5346) centre (-15.8468, -26.5346) ccw
  arc A506 (-15.8468, -24.5346) -> (-15.8468, -28.5346) centre (-15.8468, -26.5346) ccw
  arc A507 (-22.4124, -28.5346) -> (-22.4124, -24.5346) centre (-22.4124, -26.5346) ccw
  arc A508 (-22.4124, -28.5346) -> (-22.4124, -24.5346) centre (-22.4124, -26.5346) ccw
  arc A509 (-22.4124, -28.5346) -> (-22.4124, -24.5346) centre (-22.4124, -26.5346) ccw
  arc A510 (-26.3463, -31.4916) -> (-26.3463, -35.4916) centre (-26.3463, -33.4916) ccw
  arc A511 (-26.3463, -31.4916) -> (-26.3463, -35.4916) centre (-26.3463, -33.4916) ccw
  arc A512 (-26.3463, -31.4916) -> (-26.3463, -35.4916) centre (-26.3463, -33.4916) ccw
  arc A513 (-26.3463, -31.4916) -> (-26.3463, -35.4916) centre (-26.3463, -33.4916) ccw
  arc A514 (-26.3463, -31.4916) -> (-26.3463, -35.4916) centre (-26.3463, -33.4916) ccw
  arc A515 (-26.3463, -31.4916) -> (-26.3463, -35.4916) centre (-26.3463, -33.4916) ccw
  line L436 (-35.8468, -28.5346) -> (-22.4124, -28.5346)
  line L437 (-35.8468, -28.5346) -> (-22.4124, -28.5346)
  line L438 (-35.8468, -28.5346) -> (-22.4124, -28.5346)
  line L439 (-35.8468, -28.5346) -> (-22.4124, -28.5346)
  line L440 (-35.8468, -28.5346) -> (-22.4124, -28.5346)
  line L441 (-35.8468, -28.5346) -> (-22.4124, -28.5346)
  line L442 (-22.4124, -24.5346) -> (-35.8468, -24.5346)
  line L443 (-22.4124, -24.5346) -> (-35.8468, -24.5346)
  line L444 (-22.4124, -24.5346) -> (-35.8468, -24.5346)
  line L445 (-22.4124, -24.5346) -> (-35.8468, -24.5346)
  line L446 (-22.4124, -24.5346) -> (-35.8468, -24.5346)
  line L447 (-22.4124, -24.5346) -> (-35.8468, -24.5346)
  line L448 (-26.3463, -35.4916) -> (-12.9119, -35.4916)
  line L449 (-12.9119, -31.4916) -> (-26.3463, -31.4916)
  line L450 (-12.9119, -31.4916) -> (-26.3463, -31.4916)
  line L451 (-26.3463, -35.4916) -> (-12.9119, -35.4916)
  line L452 (-12.9119, -31.4916) -> (-26.3463, -31.4916)
  line L453 (-12.9119, -31.4916) -> (-26.3463, -31.4916)
  line L454 (-26.3463, -35.4916) -> (-12.9119, -35.4916)
  line L455 (-12.9119, -31.4916) -> (-26.3463, -31.4916)
  line L456 (-12.9119, -31.4916) -> (-26.3463, -31.4916)
  line L457 (-26.3463, -35.4916) -> (-12.9119, -35.4916)
  line L458 (-26.3463, -35.4916) -> (-12.9119, -35.4916)
  line L459 (-26.3463, -35.4916) -> (-12.9119, -35.4916)
  arc A516 (-12.9119, -35.4916) -> (-12.9119, -31.4916) centre (-12.9119, -33.4916) ccw
  arc A517 (-46.3463, -31.4916) -> (-46.3463, -35.4916) centre (-46.3463, -33.4916) ccw
  arc A518 (-52.9119, -35.4916) -> (-52.9119, -31.4916) centre (-52.9119, -33.4916) ccw